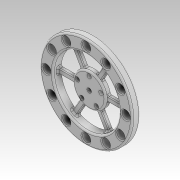
# Autodesk Inventor part: FlywheelXL
Saved by Autodesk Inventor 2020 (Build 240168000, 168)
## iProperties
Created: 2020-12-31
Part Number: FlywheelXL
Material: Generic
Document SubType Name: Modeling
Designer: DDeGo
Density: 1 g/cm^3
Appearance: Default
Author: DDeGo
Autodesk Inventor part; units mm, degrees
ref_plane "YZ Plane" through (0, 0, 0) normal (1, 0, 0) x (0, 1, 0)
ref_plane "XZ Plane" through (0, 0, 0) normal (0, 1, 0) x (-1, 0, 0)
ref_plane "XY Plane" through (0, 0, 0) normal (0, 0, 1) x (1, 0, 0)
sketch "Sketch2" plane through (0, 0, 0) normal (0, 0, 1) x (1, 0, 0)
  circle A0 centre (0, 0) radius 1.1
  circle A1 centre (0, 0) radius 10
  dimension "d46" = 20
  dimension "d47" = 2.2
  constraints: 2 centre point, 1 coincident
  measures "d46" diameter of A1
  measures "d47" diameter of A0
extrude "Extrusion2" add sketch "Sketch2" along normal blind 3
sketch "Sketch6" plane through (0, 0, 0) normal (0, 0, -1) x (-1, 0, 0)
  circle A0 centre (0, 0) radius 20
  circle A1 centre (0, 0) radius 28
  dimension "d23" = 56
  dimension "d24" = 8
  constraints: 2 centre point, 2 coincident
  measures "d23" diameter of A1
  measures "d24" radial gap between concentric circles of A0 A1
extrude "Extrusion6" add sketch "Sketch6" against normal blind 5
sketch "Sketch7" plane through (0, 0, 0) normal (0, 0, -1) x (-1, 0, 0)
  line L0 (-3.6444, 9.3123) -> (-8.6728, 18.0217)
  circle A0 centre (0, 0) radius 20 projected
  line L1 (-8.6728, 18.0217) -> (-11.2709, 16.5217) construction
  line L2 (-11.2709, 16.5217) -> (-6.2425, 7.8123)
  line L3 (-6.2425, 7.8123) -> (-3.6444, 9.3123) construction
  line L4 (0, 0) -> (0, 10) construction
  circle A1 centre (0, 0) radius 10 projected
  point P0 (-3.6444, 9.3123)
  dimension "d28" = 3
  dimension "d48" = 30
  constraints: 10 end point, 4 point on circle, 3 perpendicular, 1 vertical
  measures "d28" distance between parallel lines of L0 L2
  measures "d48" angle of L0 L4
extrude "Extrusion7" add sketch "Sketch7" against normal blind 2 contours A1 L2 A0 L0 picked at (-6.517, 11.6213)
fillet "Fillet1" radius 1 5 edges at (8.6728, 18.0217, 1) (11.2709, 16.5217, 1) (10, 17.3205, 2) (6.2425, 7.8123, 1) (3.6444, 9.3123, 1)
fillet "Fillet1" radius 0.5 2 edges at (8.7567, 12.167, 2) (6.1586, 13.667, 2)
pattern_circular "Circular Pattern1" count 6 over 360 about axis through (0, 0, 0) along (0, 0, 1) of "Extrusion7", "Fillet1"
sketch "Sketch8" plane through (0, 0, 5) normal (0, 0, 1) x (1, 0, 0)
  circle A0 centre (0, 0) radius 28 projected
  line L0 (28, 0) -> (20, 0) construction
  circle A1 centre (24, 0) radius 2.5
  circle A2 centre (0, 0) radius 20 projected
  dimension "d37" = 5
  constraints: 2 end point, 2 horizontal alignment, 1 centre point, 1 horizontal, 1 midpoint, 1 point on line, 2 other
  measures "d37" diameter of A1
extrude "Extrusion8" cut sketch "Sketch8" against normal through all contours A1
chamfer "Chamfer1" distance 0.5 angle 45 1 edges at (21.5, 0, 5)
pattern_circular "Circular Pattern2" count 12 over 360 about axis through (0, 0, 0) along (0, 0, 1) of "Extrusion8", "Chamfer1"
fillet "Fillet2" radius 1 3 edges at (20, 0, 5) (28, 0, 5) (28, 0, 0)
sketch "Sketch12" plane through (0, 0, 3) normal (0, 0, 1) x (1, 0, 0)
  line L0 (0, 12) -> (0, 3) construction
  line L1 (0, 0) -> (0, 3) construction
  circle A0 centre (0, 7.5) radius 1.35
  circle A1 centre (-7.1329, 2.3176) radius 1.35
  circle A2 centre (-4.4084, -6.0676) radius 1.35
  circle A3 centre (4.4084, -6.0676) radius 1.35
  circle A4 centre (7.1329, 2.3176) radius 1.35
  circle A5 centre (0, 0) radius 7.5 construction
  point P0 (10, 0)
  point P1 (10, 0)
  dimension "d69" = 15
  dimension "d62" = 2.7
  dimension "d65" = 360
  constraints: 5 centre point, 4 coincident, 4 end point, 1 collinear, 1 midpoint, 1 vertical, 1 vertical alignment, 13 other
  measures "d62" diameter of A0
extrude "Extrusion12" cut sketch "Sketch12" against normal through all
fillet "Fillet4" radius 1 1 edges at (-10, 0, 3)
chamfer "Chamfer3" distance 0.3 angle 45 2 edges at (-1.1, 0, 0) (-1.1, 0, 3)
body "Solid2"
